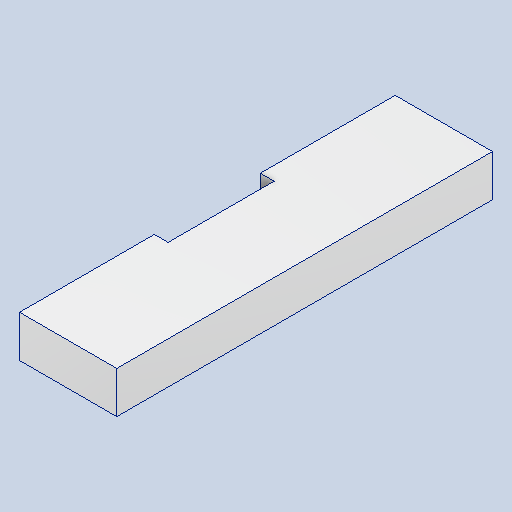
# Autodesk Inventor part: belt_liner_v2_Plate_19
Saved by Autodesk Inventor 2025.2 (Build 292293000, 293)
## iProperties
Created: 2024-12-15
Part Number: belt_liner_v2_Plate_19
Material: アルミニウム 6061
Document SubType Name: Modeling
Designer: haruy
Density: 2.7 g/cm^3
Appearance: アルミニウム - フラット
Author: haruy
Autodesk Inventor part; units mm, degrees
ref_plane "YZ Plane" through (0, 0, 0) normal (1, 0, 0) x (0, 1, 0)
ref_plane "XZ Plane" through (0, 0, 0) normal (0, 1, 0) x (-1, 0, 0)
ref_plane "XY Plane" through (0, 0, 0) normal (0, 0, 1) x (1, 0, 0)
sketch "スケッチ1" plane through (0, 0, 0) normal (1, 0, 0) x (0, 1, 0)
  line L0 (0, 0) -> (5, 0)
  line L1 (5, 0) -> (5, -45)
  line L2 (5, -45) -> (0, -45)
  line L3 (0, -45) -> (0, 0)
  circle A0 centre (2.5, -12.15) radius 1.25
  line L4 (0, -13) -> (5, -13)
  line L5 (5, -13) -> (5, -32)
  line L6 (5, -32) -> (0, -32)
  line L7 (0, -32) -> (0, -13)
  circle A1 centre (2.5, -12.15) radius 3.5
  line L8 (0, -22.5) -> (5, -22.5)
  circle A2 centre (2.5, -32.85) radius 1.25
  line L9 (5, -16.15) -> (0, -16.15)
  line L10 (0, -16.15) -> (0, -28.85)
  line L11 (0, -28.85) -> (5, -28.85)
  line L12 (5, -28.85) -> (5, -16.15)
  point P0 (5, -28.85)
  point P1 (0, -28.85)
  point P2 (0, -16.15)
  point P3 (5, -16.15)
  dimension "d0" = 5
  dimension "d1" = 45
  dimension "d2" = 2.5
  dimension "d4" = 5
  dimension "d5" = 19
  dimension "d7" = 12.15
  dimension "d8" = 2.5
  dimension "d9" = 7
  dimension "d19" = 5
  dimension "d20" = 12.7
  dimension "d21" = 6.35
  dimension "d28" = 13
  constraints: 26 end point, 6 parallel, 3 centre point, 3 horizontal, 3 perpendicular, 2 midpoint, 2 point on line, 1 coincident, 1 symmetric about line, 1 other
  measures "d0" distance of L1.end L2.end
  measures "d1" distance between parallel lines of L2 L0
  measures "d2" diameter of A0
  measures "d4" distance of L5.end L6.end
  measures "d5" distance of L4.end L5.end
  measures "d7" distance from line of A0.centre L0
  measures "d8" distance from line of A0.centre L3
  measures "d9" diameter of A1
  measures "d19" distance of L11.end L10.end
  measures "d20" distance of L10.end L9.end
  measures "d21" distance between parallel lines of L8 L9
  measures "d28" distance between parallel lines of L0 L4
extrude "押し出し1" add sketch "スケッチ1" along normal blind 10 contours L0 L1 A1 L3 | A1 L1 L4 A0 L3 | L4 A0 L1 A1 L3 | A1 L1 L9 L3 | L4 A0 | A0 L4 | L9 L1 L8 L3 | L8 L1 L11 L3 | L11 L1 L6 A2 L3 | L6 A2 L1 L2 L3 | A2 L6 | L6 A2
extrude "押し出し2" add sketch "スケッチ1" against normal blind 1.651 contours L0 L1 A1 L3 | A1 L1 L4 A0 L3 | L4 A0 L1 A1 L3 | A1 L1 L9 L3 | L11 L1 L6 A2 L3 | L6 A2 L1 L2 L3
thread "ねじ1" size "M2.5x0.45" class "6H" standard "ANSI Metric M Profile" full length
thread "ねじ2" size "M2.5x0.45" class "6H" standard "ANSI Metric M Profile" full length
